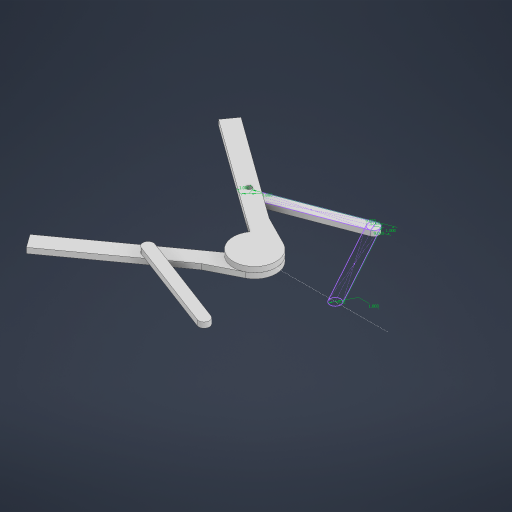
# Autodesk Inventor part: Claw
Saved by Autodesk Inventor 2023 (Build 270158000, 158)
## iProperties
Created: 2023-01-16
Part Number: Claw
Material: Generic
Document SubType Name: Modeling
Designer: Terrence
Density: 1 g/cm^3
Appearance: Default
Author: Terrence
Autodesk Inventor part; units mm, degrees
ref_plane "YZ Plane" through (0, 0, 0) normal (1, 0, 0) x (0, 1, 0)
ref_plane "XZ Plane" through (0, 0, 0) normal (0, 1, 0) x (-1, 0, 0)
ref_plane "XY Plane" through (0, 0, 0) normal (0, 0, 1) x (1, 0, 0)
sketch "Sketch1" plane through (0, 0, 0) normal (0, 1, 0) x (-1, 0, 0)
  circle A0 centre (0, 0) radius 50.8
  circle A1 centre (109, 0) radius 50.8
  line L0 (0, 0) -> (-117.0085, 0) construction
  line L1 (0, 0) -> (308.7825, -223.1913)
  line L2 (415.459, 120.65) -> (174.159, 120.65)
  line L3 (174.159, 120.65) -> (174.159, -120.65)
  line L4 (174.159, -120.65) -> (415.459, -120.65)
  line L5 (415.459, -120.65) -> (415.459, 120.65)
  line L6 (0, 0) -> (50.8, 0) construction
  line L7 (286.4634, -254.0696) -> (4.9129, -50.5619)
  line L8 (308.7825, -223.1913) -> (286.4634, -254.0696)
  line L9 (46.0839, -80.3207) -> (-22.9719, -45.3093)
  point P0 (174.159, 0)
  point P1 (41.171, -29.7588)
  point P2 (53.284, -38.5142)
  dimension "d0" = 101.6
  dimension "d1" = 101.6
  dimension "d2" = 381
  dimension "d3" = 241.3
  dimension "d4" = 241.3
  dimension "d32" = 38.1
  dimension "d33" = 50.8
  constraints: 20 end point, 4 point on line, 3 horizontal, 3 perpendicular, 3 point on circle, 2 centre point, 2 parallel, 1 coincident, 1 midpoint, 1 tangent
  measures "d0" diameter of A0
  measures "d1" diameter of A1
  measures "d2" distance of L0.start L1.end
  measures "d3" distance of L4.end L3.end
  measures "d4" distance of L3.end L2.end
  measures "d32" distance of L1.end L7.start
  measures "d33" distance of L7.end L9.start
extrude "Extrusion1" add sketch "Sketch1" along normal blind 12.7 contours A0 | A0 L7 L9 | L1 L8 L7 A0
sketch "Sketch6" plane through (0, 12.7, 0) normal (0, 1, 0) x (1, 0, 0)
  line L0 (-308.7825, 223.1913) -> (-41.171, 29.7588) projected
  line L1 (-144.0985, 104.156) -> (-121.7794, 135.0342) construction
  line L2 (-46.0839, 80.3207) -> (-286.4634, 254.0696) projected
  circle A0 centre (-132.9389, 119.5951) radius 6.35
  point P0 (0, 0)
  dimension "d34" = 127
  dimension "d35" = 12.7
  constraints: 2 end point, 2 point on line, 1 centre point, 1 midpoint, 1 perpendicular
  measures "d34" distance from line of L0.end L1
  measures "d35" diameter of A0
extrude "Extrusion7" cut sketch "Sketch6" against normal blind 12.7
sketch "Sketch7" plane through (0, 0, 0) normal (0, -1, 0) x (1, 0, 0)
  line L0 (0, 0) -> (314.9667, 0) construction
  circle A0 centre (-132.9389, -119.5951) radius 6.35 projected
  line L1 (-137.2102, -107.6349) -> (-128.6677, -131.5553) construction
  circle A1 centre (190.3953, 0) radius 12.7
  circle A2 centre (-132.9389, -119.5951) radius 12.7
  line L2 (-132.9389, -119.5951) -> (80.8179, -200.6259) construction
  line L3 (80.8179, -200.6259) -> (190.3953, 0) construction
  line L4 (-128.4372, -107.7197) -> (85.3196, -188.7505)
  line L5 (85.3196, -188.7505) -> (76.3162, -212.5012)
  line L6 (76.3162, -212.5012) -> (-137.4406, -131.4705)
  line L7 (-137.4406, -131.4705) -> (-128.4372, -107.7197)
  line L8 (-128.4372, -107.7197) -> (76.3162, -212.5012) construction
  line L9 (85.3196, -188.7505) -> (-137.4406, -131.4705) construction
  line L10 (179.2495, 6.0876) -> (69.672, -194.5382)
  line L11 (69.672, -194.5382) -> (91.9638, -206.7135) construction
  line L12 (91.9638, -206.7135) -> (201.5412, -6.0876)
  line L13 (201.5412, -6.0876) -> (179.2495, 6.0876) construction
  line L14 (179.2495, 6.0876) -> (91.9638, -206.7135) construction
  line L15 (75.4906, -186.2231) -> (201.5412, -6.0876) construction
  circle A3 centre (80.8179, -200.6259) radius 12.7
  point P0 (-26.0605, -160.1105)
  point P1 (135.6066, -100.3129)
  dimension "d39" = 25.4
  dimension "d40" = 25.4
  dimension "d41" = 25.4
  dimension "d44" = 228.6
  dimension "d45" = 228.6
  dimension "d46" = 25.4
  dimension "d47" = 25.4
  constraints: 32 end point, 6 midpoint, 6 parallel, 3 point on line, 2 centre point, 2 coincident, 2 perpendicular, 1 horizontal, 4 other
  measures "d39" distance of L1.end L1.start
  measures "d40" diameter of A1
  measures "d41" diameter of A2
  measures "d44" distance of L2.start L2.end
  measures "d45" distance of L2.end L3.end
  measures "d46" distance of L4.end L5.end
  measures "d47" distance of L11.end L10.end
extrude "Extrusion8" add sketch "Sketch7" along normal blind 12.7 separate body contours A0 L7 | A0 L7 A2 | L7 A0 | A0 L7 A2 | L4 L10 A3 L6 A2 | L4 A3 L10 | A3 L5 | L5 A3
mirror "Mirror4" about plane through (0, 0, 0) normal (0, 1, 0) bodies 1 2 separate body
mirror "Mirror6" about plane through (0, 0, 0) normal (0, 0, 1) remove original yes bodies 3 4
body "Solid1"
body "Solid5"
body "Solid6"
body "Solid7"
